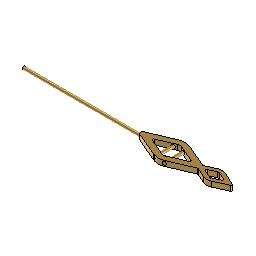
ルアンメェイ_かんざし_mk1 v4 (Autodesk Fusion 360 design; units mm, degrees)
Autodesk Fusion 360 part; units mm, degrees
sketch "スケッチ1" plane through (0, 0, 0) normal (0, 0, 1) x (1, 0, 0)
  line L0 (0, 0) -> (210, 0) construction
  dimension "d1" = 210
  constraint coincident L0.start origin
  constraint horizontal L0
  measures "d1" distance of L0.start L0.end
sketch "スケッチ1 (2)" plane through (0, 0, 0) normal (0, 0, 1) x (1, 0, 0) in component "decoration"
  line L0 (0, 0) -> (93, 0) construction
  line L1 (33, 14.25) -> (33, -8.5) construction
  line L2 (13, 0) -> (33, 8.5)
  line L3 (13, 0) -> (33, -8.5)
  line L4 (53, 0) -> (33, 8.5)
  line L5 (53, 0) -> (33, -8.5)
  line L6 (3, 0) -> (3, 1.5)
  line L7 (3, 1.5) -> (33, 14.25)
  line L8 (74.3889, 8.375) -> (74.3889, -4.5) construction
  line L9 (64.3889, 0) -> (74.3889, 4.5)
  line L10 (64.3889, 0) -> (74.3889, -4.5)
  line L11 (84.3889, 0) -> (74.3889, 4.5)
  line L12 (84.3889, 0) -> (74.3889, -4.5)
  line L13 (33, 14.25) -> (61, 2.35)
  line L14 (61, 0) -> (61, 2.35) construction
  line L15 (61, 2.35) -> (74.3889, 8.375)
  line L16 (74.3889, 8.375) -> (93, 0)
  line L17 (3, 0) -> (3, -1.5)
  line L18 (3, -1.5) -> (33, -14.25)
  line L19 (33, -14.25) -> (61, -2.35)
  line L20 (61, -2.35) -> (74.3889, -8.375)
  line L21 (74.3889, -8.375) -> (93, 0)
  dimension "d4" = 93
  dimension "d5" = 17
  dimension "d6" = 13
  dimension "d7" = 20
  dimension "d8" = 1.5
  dimension "d9" = 3
  dimension "d10" = 9
  dimension "d12" = 10
  dimension "d14" = 8
  constraint coincident L0.start origin
  constraint horizontal L0
  constraint perpendicular L0 L1
  constraint coincident L0 L2.start
  constraint symmetric L0 L2 L3
  constraint symmetric L2.end L1 L4.end
  constraint symmetric L3.end L1 L5.end
  constraint symmetric L1 L2.start L4.start
  constraint coincident L2.end L1
  constraint coincident L0 L6.start
  constraint perpendicular L0 L6
  constraint parallel L2 L7
  constraint perpendicular L0 L8
  constraint coincident L0 L9.start
  constraint symmetric L0 L9 L10
  constraint symmetric L9.end L8 L11.end
  constraint symmetric L10.end L8 L12.end
  constraint symmetric L8 L9.start L11.start
  constraint parallel L4 L13
  constraint coincident L0 L14.start
  constraint perpendicular L0 L14
  constraint parallel L9 L15
  constraint coincident L9.end L8
  constraint parallel L11 L16
  constraint coincident L0.end L16.end
  constraint symmetric L0 L6.start L17.start
  constraint symmetric L0 L6.end L17.end
  constraint symmetric L0 L1.start L18.end
  constraint symmetric L0 L13.end L19.end
  constraint symmetric L0 L8.start L20.end
  constraint symmetric L0 L16.end L21.end
  measures "d4" distance of L0.start L0.end
  measures "d5" distance of L2.end L1.end
  measures "d6" distance of L0.start L2.start
  measures "d7" distance of L1 L2.start
  measures "d8" distance of L6.start L6.end
  measures "d9" distance of L0.start L6
  measures "d10" distance of L9.end L8.end
  measures "d12" distance of L8 L9.start
  measures "d14" distance of L4.start L14
extrude "押し出し2" add sketch "スケッチ1 (2)" along normal blind 5 makes body 1 in component "decoration"
fillet "フィレット1" radius 15 2 edges at (33, -14.25, 2.5) (33, 14.25, 2.5) on bodies 1 in component "decoration"
fillet "フィレット2" radius 10 2 edges at (74.3889, 8.375, 2.5) (74.3889, -8.375, 2.5) on bodies 1 in component "decoration"
fillet "フィレット3" radius 1 1 edges at (93, 0, 2.5) on bodies 1 in component "decoration"
fillet "フィレット4" radius 1 2 edges at (84.3889, 0, 2.5) (64.3889, 0, 2.5) on bodies 1 in component "decoration"
fillet "フィレット5" radius 2 2 edges at (74.3889, 4.5, 2.5) (74.3889, -4.5, 2.5) on bodies 1 in component "decoration"
fillet "フィレット6" radius 1 2 edges at (13, 0, 2.5) (53, 0, 2.5) on bodies 1 in component "decoration"
fillet "フィレット7" radius 5 2 edges at (33, 8.5, 2.5) (33, -8.5, 2.5) on bodies 1 in component "decoration"
fillet "フィレット8" radius 1 1 edges at (61, 2.35, 2.5) on bodies 1 in component "decoration"
fillet "フィレット8" radius 1 1 edges at (61, -2.35, 2.5) on bodies 1 in component "decoration"
fillet "フィレット9" radius 1 2 edges at (3, -1.5, 2.5) (3, 1.5, 2.5) on bodies 1 in component "decoration"
sketch "スケッチ4" plane through (0, 0, 0) normal (0, 1, 0) x (1, 0, 0) in component "decoration"
  line L0 (0, 0) -> (33, 0) construction
  line L1 (33, 0) -> (33, -2.5) construction
  line L2 (28, -2.5) -> (38, -2.5) construction
  circle A0 centre (28, -2.5) radius 1.5
  circle A1 centre (38, -2.5) radius 1.5
  dimension "d44" = 2.5
  dimension "d45" = 33
  dimension "d46" = 10
  dimension "d47" = 3
  dimension "d48" = 3
  constraint coincident L0.start origin
  constraint horizontal L0
  constraint perpendicular L0 L1
  constraint horizontal L2
  constraint midpoint L1.end L2
  constraint coincident L2.start A0.centre
  constraint coincident L2.end A1.centre
  measures "d44" distance of L0.end L1.end
  measures "d45" distance of L0.start L0.end
  measures "d46" distance of L2.start L2.end
  measures "d47" diameter of A0
  measures "d48" diameter of A1
extrude "押し出し3" cut sketch "スケッチ4" against normal blind 18 bodies 1 in component "decoration"
extrude "押し出し4" cut sketch "スケッチ4" along normal blind 22 bodies 1 in component "decoration"
extrude "押し出し1" add sketch "スケッチ4" along normal up to surface separate body contours A0 end surface through (3, -1.5, 0) normal (-0.391141, -0.920331, 0) offset 0 makes body 2 in component "center piller"
extrude "押し出し2'" add sketch "スケッチ4" along normal up to surface separate body contours A1 end surface through (33, -14.25, 0) normal (0.391141, -0.920331, 0) offset 0 makes body 3 in component "center piller"
extrude "押し出し3'" add sketch "スケッチ4" along normal up to surface contours A0 end surface through (3, 1.5, 0) normal (-0.391141, 0.920331, 0) offset 0 bodies 2 in component "center piller"
extrude "押し出し4'" add sketch "スケッチ4" along normal up to surface contours A1 end surface through (33, 14.25, 0) normal (0.391141, 0.920331, 0) offset 0 bodies 3 in component "center piller"
sketch "スケッチ5" plane through (0, 0, 0) normal (1, 0, 0) x (0, 1, 0) in component "decoration"
  line L0 (0, 0) -> (0, 2.5) construction
  circle A0 centre (0, 2.5) radius 1.5
  dimension "d61" = 2.5
  dimension "d62" = 3
  constraint coincident L0.start origin
  constraint vertical L0
  constraint coincident L0.end A0.centre
  measures "d61" distance of L0.start L0.end
  measures "d62" diameter of A0
extrude "押し出し5" cut sketch "スケッチ5" along normal blind 10 bodies 1 in component "decoration"
extrude "押し出し1'" add 1 faces at (10, 0.4297, 2.7088) along direction (-1, 0, 0) blind 120 separate body on bodies 1 makes body 4 in component "pin"
component "decoration" placed x (1, 0, 0) y (0, 1, 0) z (0, 0, 1) at (0, 0, 0)
component "center piller" placed x (1, 0, 0) y (0, 1, 0) z (0, 0, 1) at (0, 0, 0)
component "pin" placed x (1, 0, 0) y (0, 1, 0) z (0, 0, 1) at (0, 0, 0)
